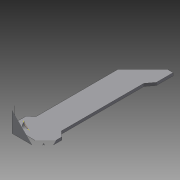
# Autodesk Inventor part: Part2
Saved by Autodesk Inventor 2014 SP1 (Build 180222100, 222)
## iProperties
Created: 2014-03-24
Part Number: Part2
Material: Generic
Document SubType Name: Modeling
Designer: tom
Density: 1 g/cm^3
Appearance: Default
Author: tom
Autodesk Inventor part; units mm, degrees
ref_plane "YZ Plane" through (0, 0, 0) normal (1, 0, 0) x (0, 1, 0)
ref_plane "XZ Plane" through (0, 0, 0) normal (0, 1, 0) x (-1, 0, 0)
ref_plane "XY Plane" through (0, 0, 0) normal (0, 0, 1) x (1, 0, 0)
ref_plane "Work Plane1" through (3.4455, 2.6204, 52.7) normal (0, 0, 1) x (1, 0, 0)
sketch "Sketch1" plane through (3.4455, 2.6204, 52.7) normal (0, 0, 1) x (1, 0, 0)
  circle A0 centre (0, 0) radius 1.5 projected
  line L0 (-5.25, 4.25) -> (5.25, 4.25)
  line L1 (5.25, 4.25) -> (5.25, -5.25)
  line L2 (5.25, -5.25) -> (-5.25, -5.25)
  line L3 (-5.25, -5.25) -> (-5.25, 4.25)
  point P0 (-3.4455, -2.6204)
  dimension "d2" = 10.5
  dimension "d4" = 4.25
  dimension "d6" = 5.25
  dimension "d7" = 9.5
  constraints: 8 end point, 3 perpendicular
  measures "d2" distance of L0.start L0.end
  measures "d4" distance from line of L0 A0.centre
  measures "d6" horizontal distance of L0.end A0.centre
  measures "d7" distance of L0.end L1.end
extrude "Extrusion1" add sketch "Sketch1" along normal blind 1.15
sketch "Sketch2" plane through (3.4455, 2.6204, 52.7) normal (0, 0, -1) x (-1, 0, 0)
  line L0 (-5.25, 4.25) -> (-5.25, -5.25) projected
  line L1 (-5.25, -5.25) -> (5.25, -5.25) projected
  line L2 (5.25, -5.25) -> (5.25, 4.25) projected
  line L3 (-5.25, -5.25) -> (-5.25, -4.1)
  line L4 (-5.25, -4.1) -> (5.25, -4.1)
  point P0 (3.4455, -2.6204)
  dimension "d10" = 1.15
  constraints: 4 end point, 2 point on line, 1 perpendicular
  measures "d10" distance of L0.end L3.end
extrude "Extrusion2" add sketch "Sketch2" along normal blind 1.5
sketch "Sketch3" plane through (-1.8045, -2.6296, 53.85) normal (0, -1, 0) x (1, 0, 0)
  line L0 (0, 0) -> (10.5, 0) projected
  line L1 (10.5, -2.65) -> (0, -2.65) projected
  line L2 (5.25, -54.5) -> (12.75, -54.5)
  line L3 (5.25, 0) -> (5.25, -54.5) construction
  line L4 (12.75, -54.5) -> (12.75, -47.5)
  line L5 (10.5, -10) -> (10.5, -44.5)
  line L6 (12.75, -2.65) -> (12.75, -8)
  line L7 (5.25, -2.65) -> (12.75, -2.65)
  line L8 (12.75, -8) -> (10.5, -10)
  line L9 (10.5, -44.5) -> (12.75, -47.5)
  line L10 (5.25, -54.5) -> (-2.25, -54.5)
  line L11 (-2.25, -54.5) -> (-2.25, -47.5)
  line L12 (0, -10) -> (0, -44.5)
  line L13 (-2.25, -2.65) -> (-2.25, -8)
  line L14 (5.25, -2.65) -> (-2.25, -2.65)
  line L15 (-2.25, -8) -> (0, -10)
  line L16 (0, -44.5) -> (-2.25, -47.5)
  circle A0 centre (5.25, -5.75) radius 1.125
  circle A1 centre (0.75, -5.75) radius 1.125
  circle A2 centre (9.75, -5.75) radius 1.125
  circle A3 centre (0.75, -49.75) radius 1.125
  circle A4 centre (9.75, -49.75) radius 1.125
  circle A5 centre (5.25, -49.75) radius 1.125
  dimension "d13" = 54.5
  dimension "d15" = 7.5
  dimension "d16" = 7
  dimension "d17" = 10
  dimension "d18" = 34.5
  dimension "d19" = 5.25
  dimension "d20" = 8
  dimension "d21" = 7.5
  dimension "d24" = 2.25
  dimension "d25" = 5.75
  dimension "d26" = 2.25
  dimension "d27" = 4.5
  dimension "d28" = 2.25
  dimension "d29" = 4.5
  dimension "d30" = 4.75
  dimension "d32" = 5.75
  dimension "d33" = 4.5
  dimension "d34" = 2.25
  dimension "d35" = 2.25
  dimension "d36" = 2.25
  constraints: 30 end point, 6 centre point, 6 symmetric about line, 4 parallel, 3 point on line, 2 midpoint, 1 perpendicular
  measures "d13" distance between parallel lines of L2 L0
  measures "d15" distance from line of L3 L2.end
  measures "d16" distance of L2.end L4.end
  measures "d17" distance from line of L2 L5.end
  measures "d18" distance of L5.start L5.end
  measures "d19" distance between parallel lines of L3 L5
  measures "d20" distance from line of L0 L6.end
  measures "d21" distance between parallel lines of L3 L6
  measures "d24" diameter of A0
  measures "d25" distance from line of L0 A0.centre
  measures "d26" diameter of A1
  measures "d27" distance of A0.centre A1.centre
  measures "d28" diameter of A2
  measures "d29" distance of A0.centre A2.centre
  measures "d30" distance from line of L10 A3.centre
  measures "d32" distance from line of L0 A1.centre
  measures "d33" distance from line of L3 A3.centre
  measures "d34" diameter of A3
  measures "d35" diameter of A4
  measures "d36" diameter of A5
extrude "Extrusion3" add sketch "Sketch3" against normal blind 1.15
sketch "Sketch4" plane through (10.9455, -2.6296, -0.65) normal (0, 0, -1) x (-1, 0, 0)
  line L0 (2.25, 1.15) -> (12.75, 1.15) projected
  line L1 (12.75, 1.15) -> (12.75, 9.5) projected
  line L2 (12.75, 9.5) -> (2.25, 9.5) projected
  line L3 (2.25, 9.5) -> (2.25, 1.15) projected
  circle A0 centre (7.5, 5.25) radius 1.5 projected
  line L4 (0, 1.15) -> (0, 5.25)
  line L5 (15, 1.15) -> (15, 5.25)
  line L6 (0, 1.15) -> (15, 1.15)
  circle A1 centre (7.5, 5.25) radius 1.5
  arc A2 (1.2199, 1.15) -> (13.7801, 1.15) centre (7.5, 5.25) ccw
  arc A3 (15, 5.25) -> (0, 5.25) centre (7.5, 5.25) ccw
  point P0 (10.9455, 2.6296)
  constraints: 6 end point, 4 point on circle, 3 centre point, 2 coincident, 2 point on line, 1 concentric, 1 parallel, 1 tangent
extrude "Extrusion4" add sketch "Sketch4" against normal blind 1.15 contours L3 L2 L1 L0 | L6 L4 A3 L5 L1 L2 L3
body "Solid1"
